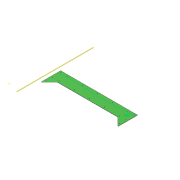
# Autodesk Inventor part: Acrylic-Side-Panel_CPY
Saved by Autodesk Inventor 2017 (Build 210142000, 142)
## iProperties
Created: 2016-07-12
Part Number: Acrylic-Side-Panel_CPY
Material: Generic
Document SubType Name: Modeling
Designer: joshmamo
Density: 1 g/cm^3
Appearance: Default
Author: joshmamo
Autodesk Inventor part; units mm, degrees
(part 1 of 3)
ref_plane "YZ Plane" through (0, 0, 0) normal (1, 0, 0) x (0, 1, 0)
ref_plane "XZ Plane" through (0, 0, 0) normal (0, 1, 0) x (-1, 0, 0)
ref_plane "XY Plane" through (0, 0, 0) normal (0, 0, 1) x (1, 0, 0)
ref_plane "Work Plane1" through (87.4375, 600, -660) normal (0, 0, -1) x (1, 0, 0)
sketch "Sketch1" plane through (87.4375, 600, -660) normal (0, 0, -1) x (1, 0, 0)
  line L0 (35.8425, 447.4613) -> (35.8425, 283.4613)
  line L1 (35.8425, 283.4613) -> (695.8425, 283.4613)
  line L2 (695.8425, 283.4613) -> (695.8425, 447.4613)
  line L3 (695.8425, 447.4613) -> (695.8027, 447.8653)
  line L4 (695.8027, 447.8653) -> (695.6848, 448.2538)
  line L5 (695.6848, 448.2538) -> (695.4935, 448.6119)
  line L6 (695.4935, 448.6119) -> (695.2359, 448.9257)
  line L7 (695.2359, 448.9257) -> (694.9221, 449.1833)
  line L8 (694.9221, 449.1833) -> (694.564, 449.3747)
  line L9 (694.564, 449.3747) -> (694.1755, 449.4925)
  line L10 (694.1755, 449.4925) -> (693.7714, 449.5323)
  line L11 (693.7714, 449.5323) -> (693.3674, 449.4925)
  line L12 (693.3674, 449.4925) -> (692.9789, 449.3747)
  line L13 (692.9789, 449.3747) -> (692.6208, 449.1833)
  line L14 (692.6208, 449.1833) -> (692.307, 448.9257)
  line L15 (692.307, 448.9257) -> (625.8425, 382.4613)
  line L16 (625.8425, 382.4613) -> (105.8425, 382.4613)
  line L17 (105.8425, 382.4613) -> (39.378, 448.9257)
  line L18 (39.378, 448.9257) -> (39.0642, 449.1833)
  line L19 (39.0642, 449.1833) -> (38.7061, 449.3747)
  line L20 (38.7061, 449.3747) -> (38.3176, 449.4925)
  line L21 (38.3176, 449.4925) -> (37.9136, 449.5323)
  line L22 (37.9136, 449.5323) -> (37.5095, 449.4925)
  line L23 (37.5095, 449.4925) -> (37.121, 449.3747)
  line L24 (37.121, 449.3747) -> (36.7629, 449.1833)
  line L25 (36.7629, 449.1833) -> (36.4491, 448.9257)
  line L26 (36.4491, 448.9257) -> (36.1915, 448.6119)
  line L27 (36.1915, 448.6119) -> (36.0002, 448.2538)
  line L28 (36.0002, 448.2538) -> (35.8823, 447.8653)
  line L29 (35.8823, 447.8653) -> (35.8425, 447.4613)
  line L30 (678.4084, 421.8091) -> (678.3225, 422.4613)
  line L31 (678.3225, 422.4613) -> (678.4084, 423.1135)
  line L32 (678.4084, 423.1135) -> (678.6601, 423.7213)
  line L33 (678.6601, 423.7213) -> (679.0606, 424.2432)
  line L34 (679.0606, 424.2432) -> (679.5825, 424.6437)
  line L35 (679.5825, 424.6437) -> (680.1903, 424.8954)
  line L36 (680.1903, 424.8954) -> (680.8425, 424.9813)
  line L37 (680.8425, 424.9813) -> (681.4947, 424.8954)
  line L38 (681.4947, 424.8954) -> (682.1025, 424.6437)
  line L39 (682.1025, 424.6437) -> (682.6244, 424.2432)
  line L40 (682.6244, 424.2432) -> (683.0249, 423.7213)
  line L41 (683.0249, 423.7213) -> (683.2766, 423.1135)
  line L42 (683.2766, 423.1135) -> (683.3625, 422.4613)
  line L43 (683.3625, 422.4613) -> (683.2766, 421.8091)
  line L44 (683.2766, 421.8091) -> (683.0249, 421.2013)
  line L45 (683.0249, 421.2013) -> (682.6244, 420.6794)
  line L46 (682.6244, 420.6794) -> (682.1025, 420.2789)
  line L47 (682.1025, 420.2789) -> (681.4947, 420.0271)
  line L48 (681.4947, 420.0271) -> (680.8425, 419.9413)
  line L49 (680.8425, 419.9413) -> (680.1903, 420.0271)
  line L50 (680.1903, 420.0271) -> (679.5825, 420.2789)
  line L51 (679.5825, 420.2789) -> (679.0606, 420.6794)
  line L52 (679.0606, 420.6794) -> (678.6601, 421.2013)
  line L53 (678.6601, 421.2013) -> (678.4084, 421.8091)
  line L54 (103.6601, 368.7213) -> (104.0606, 369.2432)
  line L55 (104.0606, 369.2432) -> (104.5825, 369.6437)
  line L56 (104.5825, 369.6437) -> (105.1903, 369.8954)
  line L57 (105.1903, 369.8954) -> (105.8425, 369.9813)
  line L58 (105.8425, 369.9813) -> (106.4947, 369.8954)
  line L59 (106.4947, 369.8954) -> (107.1025, 369.6437)
  line L60 (107.1025, 369.6437) -> (107.6244, 369.2432)
  line L61 (107.6244, 369.2432) -> (108.0249, 368.7213)
  line L62 (108.0249, 368.7213) -> (108.2766, 368.1135)
  line L63 (108.2766, 368.1135) -> (108.3625, 367.4613)
  line L64 (108.3625, 367.4613) -> (108.2766, 366.8091)
  line L65 (108.2766, 366.8091) -> (108.0249, 366.2013)
  line L66 (108.0249, 366.2013) -> (107.6244, 365.6794)
  line L67 (107.6244, 365.6794) -> (107.1025, 365.2789)
  line L68 (107.1025, 365.2789) -> (106.4947, 365.0271)
  line L69 (106.4947, 365.0271) -> (105.8425, 364.9413)
  line L70 (105.8425, 364.9413) -> (105.1903, 365.0271)
  line L71 (105.1903, 365.0271) -> (104.5825, 365.2789)
  line L72 (104.5825, 365.2789) -> (104.0606, 365.6794)
  line L73 (104.0606, 365.6794) -> (103.6601, 366.2013)
  line L74 (103.6601, 366.2013) -> (103.4084, 366.8091)
  line L75 (103.4084, 366.8091) -> (103.3225, 367.4613)
  line L76 (103.3225, 367.4613) -> (103.4084, 368.1135)
  line L77 (103.4084, 368.1135) -> (103.6601, 368.7213)
  line L78 (235.1106, 369.2432) -> (235.6325, 369.6437)
  line L79 (235.6325, 369.6437) -> (236.2403, 369.8954)
  line L80 (236.2403, 369.8954) -> (236.8925, 369.9813)
  line L81 (236.8925, 369.9813) -> (237.5447, 369.8954)
  line L82 (237.5447, 369.8954) -> (238.1525, 369.6437)
  line L83 (238.1525, 369.6437) -> (238.6744, 369.2432)
  line L84 (238.6744, 369.2432) -> (239.0749, 368.7213)
  line L85 (239.0749, 368.7213) -> (239.3266, 368.1135)
  line L86 (239.3266, 368.1135) -> (239.4125, 367.4613)
  line L87 (239.4125, 367.4613) -> (239.3266, 366.8091)
  line L88 (239.3266, 366.8091) -> (239.0749, 366.2013)
  line L89 (239.0749, 366.2013) -> (238.6744, 365.6794)
  line L90 (238.6744, 365.6794) -> (238.1525, 365.2789)
  line L91 (238.1525, 365.2789) -> (237.5447, 365.0271)
  line L92 (237.5447, 365.0271) -> (236.8925, 364.9413)
  line L93 (236.8925, 364.9413) -> (236.2403, 365.0271)
  line L94 (236.2403, 365.0271) -> (235.6325, 365.2789)
  line L95 (235.6325, 365.2789) -> (235.1106, 365.6794)
  line L96 (235.1106, 365.6794) -> (234.7101, 366.2013)
  line L97 (234.7101, 366.2013) -> (234.4584, 366.8091)
  line L98 (234.4584, 366.8091) -> (234.3725, 367.4613)
  line L99 (234.3725, 367.4613) -> (234.4584, 368.1135)
  line L100 (234.4584, 368.1135) -> (234.7101, 368.7213)
  line L101 (234.7101, 368.7213) -> (235.1106, 369.2432)
  line L102 (363.4084, 366.8091) -> (363.3225, 367.4613)
  line L103 (363.3225, 367.4613) -> (363.4084, 368.1135)
  line L104 (363.4084, 368.1135) -> (363.6601, 368.7213)
  line L105 (363.6601, 368.7213) -> (364.0606, 369.2432)
  line L106 (364.0606, 369.2432) -> (364.5825, 369.6437)
  line L107 (364.5825, 369.6437) -> (365.1903, 369.8954)
  line L108 (365.1903, 369.8954) -> (365.8425, 369.9813)
  line L109 (365.8425, 369.9813) -> (366.4947, 369.8954)
  line L110 (366.4947, 369.8954) -> (367.1025, 369.6437)
  line L111 (367.1025, 369.6437) -> (367.6244, 369.2432)
  line L112 (367.6244, 369.2432) -> (368.0249, 368.7213)
  line L113 (368.0249, 368.7213) -> (368.2766, 368.1135)
  line L114 (368.2766, 368.1135) -> (368.3625, 367.4613)
  line L115 (368.3625, 367.4613) -> (368.2766, 366.8091)
  line L116 (368.2766, 366.8091) -> (368.0249, 366.2013)
  line L117 (368.0249, 366.2013) -> (367.6244, 365.6794)
  line L118 (367.6244, 365.6794) -> (367.1025, 365.2789)
  line L119 (367.1025, 365.2789) -> (366.4947, 365.0271)
  line L120 (366.4947, 365.0271) -> (365.8425, 364.9413)
  line L121 (365.8425, 364.9413) -> (365.1903, 365.0271)
  line L122 (365.1903, 365.0271) -> (364.5825, 365.2789)
  line L123 (364.5825, 365.2789) -> (364.0606, 365.6794)
  line L124 (364.0606, 365.6794) -> (363.6601, 366.2013)
  line L125 (363.6601, 366.2013) -> (363.4084, 366.8091)
  line L126 (492.3584, 366.8091) -> (492.2725, 367.4613)
  line L127 (492.2725, 367.4613) -> (492.3584, 368.1135)
  line L128 (492.3584, 368.1135) -> (492.6101, 368.7213)
  line L129 (492.6101, 368.7213) -> (493.0106, 369.2432)
  line L130 (493.0106, 369.2432) -> (493.5325, 369.6437)
  line L131 (493.5325, 369.6437) -> (494.1403, 369.8954)
  line L132 (494.1403, 369.8954) -> (494.7925, 369.9813)
  line L133 (494.7925, 369.9813) -> (495.4447, 369.8954)
  line L134 (495.4447, 369.8954) -> (496.0525, 369.6437)
  line L135 (496.0525, 369.6437) -> (496.5744, 369.2432)
  line L136 (496.5744, 369.2432) -> (496.9749, 368.7213)
  line L137 (496.9749, 368.7213) -> (497.2266, 368.1135)
  line L138 (497.2266, 368.1135) -> (497.3125, 367.4613)
  line L139 (497.3125, 367.4613) -> (497.2266, 366.8091)
  line L140 (497.2266, 366.8091) -> (496.9749, 366.2013)
  line L141 (496.9749, 366.2013) -> (496.5744, 365.6794)
  line L142 (496.5744, 365.6794) -> (496.0525, 365.2789)
  line L143 (496.0525, 365.2789) -> (495.4447, 365.0271)
  line L144 (495.4447, 365.0271) -> (494.7925, 364.9413)
  line L145 (494.7925, 364.9413) -> (494.1403, 365.0271)
  line L146 (494.1403, 365.0271) -> (493.5325, 365.2789)
  line L147 (493.5325, 365.2789) -> (493.0106, 365.6794)
  line L148 (493.0106, 365.6794) -> (492.6101, 366.2013)
  line L149 (492.6101, 366.2013) -> (492.3584, 366.8091)
  line L150 (48.4084, 296.809) -> (48.3225, 297.4613)
  line L151 (48.3225, 297.4613) -> (48.4084, 298.1135)
  line L152 (48.4084, 298.1135) -> (48.6601, 298.7212)
  line L153 (48.6601, 298.7212) -> (49.0606, 299.2432)
  line L154 (49.0606, 299.2432) -> (49.5825, 299.6437)
  line L155 (49.5825, 299.6437) -> (50.1903, 299.8954)
  line L156 (50.1903, 299.8954) -> (50.8425, 299.9813)
  line L157 (50.8425, 299.9813) -> (51.4947, 299.8954)
  line L158 (51.4947, 299.8954) -> (52.1025, 299.6437)
  line L159 (52.1025, 299.6437) -> (52.6244, 299.2432)
  line L160 (52.6244, 299.2432) -> (53.0249, 298.7212)
  line L161 (53.0249, 298.7212) -> (53.2766, 298.1135)
  line L162 (53.2766, 298.1135) -> (53.3625, 297.4613)
  line L163 (53.3625, 297.4613) -> (53.2766, 296.809)
  line L164 (53.2766, 296.809) -> (53.0249, 296.2012)
  line L165 (53.0249, 296.2012) -> (52.6244, 295.6793)
  line L166 (52.6244, 295.6793) -> (52.1025, 295.2789)
  line L167 (52.1025, 295.2789) -> (51.4947, 295.0271)
  line L168 (51.4947, 295.0271) -> (50.8425, 294.9413)
  line L169 (50.8425, 294.9413) -> (50.1903, 295.0271)
  line L170 (50.1903, 295.0271) -> (49.5825, 295.2789)
  line L171 (49.5825, 295.2789) -> (49.0606, 295.6793)
  line L172 (49.0606, 295.6793) -> (48.6601, 296.2012)
  line L173 (48.6601, 296.2012) -> (48.4084, 296.809)
  line L174 (48.4084, 366.8091) -> (48.3225, 367.4613)
  line L175 (48.3225, 367.4613) -> (48.4084, 368.1135)
  line L176 (48.4084, 368.1135) -> (48.6601, 368.7213)
  line L177 (48.6601, 368.7213) -> (49.0606, 369.2432)
  line L178 (49.0606, 369.2432) -> (49.5825, 369.6437)
  line L179 (49.5825, 369.6437) -> (50.1903, 369.8954)
  line L180 (50.1903, 369.8954) -> (50.8425, 369.9813)
  line L181 (50.8425, 369.9813) -> (51.4947, 369.8954)
  line L182 (51.4947, 369.8954) -> (52.1025, 369.6437)
  line L183 (52.1025, 369.6437) -> (52.6244, 369.2432)
  line L184 (52.6244, 369.2432) -> (53.0249, 368.7213)
  line L185 (53.0249, 368.7213) -> (53.2766, 368.1135)
  line L186 (53.2766, 368.1135) -> (53.3625, 367.4613)
  line L187 (53.3625, 367.4613) -> (53.2766, 366.8091)
  line L188 (53.2766, 366.8091) -> (53.0249, 366.2013)
  line L189 (53.0249, 366.2013) -> (52.6244, 365.6794)
  line L190 (52.6244, 365.6794) -> (52.1025, 365.2789)
  line L191 (52.1025, 365.2789) -> (51.4947, 365.0271)
  line L192 (51.4947, 365.0271) -> (50.8425, 364.9413)
  line L193 (50.8425, 364.9413) -> (50.1903, 365.0271)
  line L194 (50.1903, 365.0271) -> (49.5825, 365.2789)
  line L195 (49.5825, 365.2789) -> (49.0606, 365.6794)
  line L196 (49.0606, 365.6794) -> (48.6601, 366.2013)
  line L197 (48.6601, 366.2013) -> (48.4084, 366.8091)
  line L198 (48.4084, 421.8091) -> (48.3225, 422.4613)
  line L199 (48.3225, 422.4613) -> (48.4084, 423.1135)
  line L200 (48.4084, 423.1135) -> (48.6601, 423.7213)
  line L201 (48.6601, 423.7213) -> (49.0606, 424.2432)
  line L202 (49.0606, 424.2432) -> (49.5825, 424.6437)
  line L203 (49.5825, 424.6437) -> (50.1903, 424.8954)
  line L204 (50.1903, 424.8954) -> (50.8425, 424.9813)
  line L205 (50.8425, 424.9813) -> (51.4947, 424.8954)
  line L206 (51.4947, 424.8954) -> (52.1025, 424.6437)
  line L207 (52.1025, 424.6437) -> (52.6244, 424.2432)
  line L208 (52.6244, 424.2432) -> (53.0249, 423.7213)
  line L209 (53.0249, 423.7213) -> (53.2766, 423.1135)
  line L210 (53.2766, 423.1135) -> (53.3625, 422.4613)
  line L211 (53.3625, 422.4613) -> (53.2766, 421.8091)
  line L212 (53.2766, 421.8091) -> (53.0249, 421.2013)
  line L213 (53.0249, 421.2013) -> (52.6244, 420.6794)
  line L214 (52.6244, 420.6794) -> (52.1025, 420.2789)
  line L215 (52.1025, 420.2789) -> (51.4947, 420.0271)
  line L216 (51.4947, 420.0271) -> (50.8425, 419.9413)
  line L217 (50.8425, 419.9413) -> (50.1903, 420.0271)
  line L218 (50.1903, 420.0271) -> (49.5825, 420.2789)
  line L219 (49.5825, 420.2789) -> (49.0606, 420.6794)
  line L220 (49.0606, 420.6794) -> (48.6601, 421.2013)
  line L221 (48.6601, 421.2013) -> (48.4084, 421.8091)
  line L222 (678.4084, 366.8091) -> (678.3225, 367.4613)
  line L223 (678.3225, 367.4613) -> (678.4084, 368.1135)
  line L224 (678.4084, 368.1135) -> (678.6601, 368.7213)
  line L225 (678.6601, 368.7213) -> (679.0606, 369.2432)
  line L226 (679.0606, 369.2432) -> (679.5825, 369.6437)
  line L227 (679.5825, 369.6437) -> (680.1903, 369.8954)
  line L228 (680.1903, 369.8954) -> (680.8425, 369.9813)
  line L229 (680.8425, 369.9813) -> (681.4947, 369.8954)
  line L230 (681.4947, 369.8954) -> (682.1025, 369.6437)
  line L231 (682.1025, 369.6437) -> (682.6244, 369.2432)
  line L232 (682.6244, 369.2432) -> (683.0249, 368.7213)
  line L233 (683.0249, 368.7213) -> (683.2766, 368.1135)
  line L234 (683.2766, 368.1135) -> (683.3625, 367.4613)
  line L235 (683.3625, 367.4613) -> (683.2766, 366.8091)
  line L236 (683.2766, 366.8091) -> (683.0249, 366.2013)
  line L237 (683.0249, 366.2013) -> (682.6244, 365.6794)
  line L238 (682.6244, 365.6794) -> (682.1025, 365.2789)
  line L239 (682.1025, 365.2789) -> (681.4947, 365.0271)
  line L240 (681.4947, 365.0271) -> (680.8425, 364.9413)
  line L241 (680.8425, 364.9413) -> (680.1903, 365.0271)
  line L242 (680.1903, 365.0271) -> (679.5825, 365.2789)
  line L243 (679.5825, 365.2789) -> (679.0606, 365.6794)
  line L244 (679.0606, 365.6794) -> (678.6601, 366.2013)
  line L245 (678.6601, 366.2013) -> (678.4084, 366.8091)
  line L246 (680.1903, 295.0271) -> (679.5825, 295.2789)
  line L247 (679.5825, 295.2789) -> (679.0606, 295.6793)
  line L248 (679.0606, 295.6793) -> (678.6601, 296.2012)
  line L249 (678.6601, 296.2012) -> (678.4084, 296.809)
  line L250 (678.4084, 296.809) -> (678.3225, 297.4613)
  line L251 (678.3225, 297.4613) -> (678.4084, 298.1135)
  line L252 (678.4084, 298.1135) -> (678.6601, 298.7212)
  line L253 (678.6601, 298.7212) -> (679.0606, 299.2432)
  line L254 (679.0606, 299.2432) -> (679.5825, 299.6437)
  line L255 (679.5825, 299.6437) -> (680.1903, 299.8954)
  line L256 (680.1903, 299.8954) -> (680.8425, 299.9813)
  line L257 (680.8425, 299.9813) -> (681.4947, 299.8954)
  line L258 (681.4947, 299.8954) -> (682.1025, 299.6437)
  line L259 (682.1025, 299.6437) -> (682.6244, 299.2432)
  line L260 (682.6244, 299.2432) -> (683.0249, 298.7212)
  line L261 (683.0249, 298.7212) -> (683.2766, 298.1135)
  line L262 (683.2766, 298.1135) -> (683.3625, 297.4613)
  line L263 (683.3625, 297.4613) -> (683.2766, 296.809)
  line L264 (683.2766, 296.809) -> (683.0249, 296.2012)
  line L265 (683.0249, 296.2012) -> (682.6244, 295.6793)
  line L266 (682.6244, 295.6793) -> (682.1025, 295.2789)
  line L267 (682.1025, 295.2789) -> (681.4947, 295.0271)
  line L268 (681.4947, 295.0271) -> (680.8425, 294.9413)
  line L269 (680.8425, 294.9413) -> (680.1903, 295.0271)
  line L270 (623.4084, 296.809) -> (623.3225, 297.4613)
  line L271 (623.3225, 297.4613) -> (623.4084, 298.1135)
  line L272 (623.4084, 298.1135) -> (623.6601, 298.7212)
  line L273 (623.6601, 298.7212) -> (624.0606, 299.2432)
  line L274 (624.0606, 299.2432) -> (624.5825, 299.6437)
  line L275 (624.5825, 299.6437) -> (625.1903, 299.8954)
  line L276 (625.1903, 299.8954) -> (625.8425, 299.9813)
  line L277 (625.8425, 299.9813) -> (626.4947, 299.8954)
  line L278 (626.4947, 299.8954) -> (627.1025, 299.6437)
  line L279 (627.1025, 299.6437) -> (627.6244, 299.2432)
  line L280 (627.6244, 299.2432) -> (628.0249, 298.7212)
  line L281 (628.0249, 298.7212) -> (628.2766, 298.1135)
  line L282 (628.2766, 298.1135) -> (628.3625, 297.4613)
  line L283 (628.3625, 297.4613) -> (628.2766, 296.809)
  line L284 (628.2766, 296.809) -> (628.0249, 296.2012)
  line L285 (628.0249, 296.2012) -> (627.6244, 295.6793)
  line L286 (627.6244, 295.6793) -> (627.1025, 295.2789)
  line L287 (627.1025, 295.2789) -> (626.4947, 295.0271)
  line L288 (626.4947, 295.0271) -> (625.8425, 294.9413)
  line L289 (625.8425, 294.9413) -> (625.1903, 295.0271)
  line L290 (625.1903, 295.0271) -> (624.5825, 295.2789)
  line L291 (624.5825, 295.2789) -> (624.0606, 295.6793)
  line L292 (624.0606, 295.6793) -> (623.6601, 296.2012)
  line L293 (623.6601, 296.2012) -> (623.4084, 296.809)
  line L294 (623.4084, 366.8091) -> (623.3225, 367.4613)
  line L295 (623.3225, 367.4613) -> (623.4084, 368.1135)
  line L296 (623.4084, 368.1135) -> (623.6601, 368.7213)
  line L297 (623.6601, 368.7213) -> (624.0606, 369.2432)
  line L298 (624.0606, 369.2432) -> (624.5825, 369.6437)
  line L299 (624.5825, 369.6437) -> (625.1903, 369.8954)
  line L300 (625.1903, 369.8954) -> (625.8425, 369.9813)
  line L301 (625.8425, 369.9813) -> (626.4947, 369.8954)
  line L302 (626.4947, 369.8954) -> (627.1025, 369.6437)
  line L303 (627.1025, 369.6437) -> (627.6244, 369.2432)
  line L304 (627.6244, 369.2432) -> (628.0249, 368.7213)
  line L305 (628.0249, 368.7213) -> (628.2766, 368.1135)
  line L306 (628.2766, 368.1135) -> (628.3625, 367.4613)
  line L307 (628.3625, 367.4613) -> (628.2766, 366.8091)
  line L308 (628.2766, 366.8091) -> (628.0249, 366.2013)
  line L309 (628.0249, 366.2013) -> (627.6244, 365.6794)
  line L310 (627.6244, 365.6794) -> (627.1025, 365.2789)
  line L311 (627.1025, 365.2789) -> (626.4947, 365.0271)
  line L312 (626.4947, 365.0271) -> (625.8425, 364.9413)
  line L313 (625.8425, 364.9413) -> (625.1903, 365.0271)
  line L314 (625.1903, 365.0271) -> (624.5825, 365.2789)
  line L315 (624.5825, 365.2789) -> (624.0606, 365.6794)
  line L316 (624.0606, 365.6794) -> (623.6601, 366.2013)
  line L317 (623.6601, 366.2013) -> (623.4084, 366.8091)
  line L318 (492.3584, 296.809) -> (492.2725, 297.4613)
  line L319 (492.2725, 297.4613) -> (492.3584, 298.1135)
  line L320 (492.3584, 298.1135) -> (492.6101, 298.7212)
  line L321 (492.6101, 298.7212) -> (493.0106, 299.2432)
  line L322 (493.0106, 299.2432) -> (493.5325, 299.6437)
  line L323 (493.5325, 299.6437) -> (494.1403, 299.8954)
  line L324 (494.1403, 299.8954) -> (494.7925, 299.9813)
  line L325 (494.7925, 299.9813) -> (495.4447, 299.8954)
  line L326 (495.4447, 299.8954) -> (496.0525, 299.6437)
  line L327 (496.0525, 299.6437) -> (496.5744, 299.2432)
  line L328 (496.5744, 299.2432) -> (496.9749, 298.7212)
  line L329 (496.9749, 298.7212) -> (497.2266, 298.1135)
  line L330 (497.2266, 298.1135) -> (497.3125, 297.4613)
  line L331 (497.3125, 297.4613) -> (497.2266, 296.809)
  line L332 (497.2266, 296.809) -> (496.9749, 296.2012)
  line L333 (496.9749, 296.2012) -> (496.5744, 295.6793)
  line L334 (496.5744, 295.6793) -> (496.0525, 295.2789)
  line L335 (496.0525, 295.2789) -> (495.4447, 295.0271)
  line L336 (495.4447, 295.0271) -> (494.7925, 294.9413)
  line L337 (494.7925, 294.9413) -> (494.1403, 295.0271)
  line L338 (494.1403, 295.0271) -> (493.5325, 295.2789)
  line L339 (493.5325, 295.2789) -> (493.0106, 295.6793)
  line L340 (493.0106, 295.6793) -> (492.6101, 296.2012)
  line L341 (492.6101, 296.2012) -> (492.3584, 296.809)
  line L342 (363.4084, 296.809) -> (363.3225, 297.4613)
  line L343 (363.3225, 297.4613) -> (363.4084, 298.1135)
  line L344 (363.4084, 298.1135) -> (363.6601, 298.7212)
  line L345 (363.6601, 298.7212) -> (364.0606, 299.2432)
  line L346 (364.0606, 299.2432) -> (364.5825, 299.6437)
  line L347 (364.5825, 299.6437) -> (365.1903, 299.8954)
  line L348 (365.1903, 299.8954) -> (365.8425, 299.9813)
  line L349 (365.8425, 299.9813) -> (366.4947, 299.8954)
  line L350 (366.4947, 299.8954) -> (367.1025, 299.6437)
  line L351 (367.1025, 299.6437) -> (367.6244, 299.2432)
  line L352 (367.6244, 299.2432) -> (368.0249, 298.7212)
  line L353 (368.0249, 298.7212) -> (368.2766, 298.1135)
  line L354 (368.2766, 298.1135) -> (368.3625, 297.4613)
  line L355 (368.3625, 297.4613) -> (368.2766, 296.809)
  line L356 (368.2766, 296.809) -> (368.0249, 296.2012)
  line L357 (368.0249, 296.2012) -> (367.6244, 295.6793)
  line L358 (367.6244, 295.6793) -> (367.1025, 295.2789)
  line L359 (367.1025, 295.2789) -> (366.4947, 295.0271)
  line L360 (366.4947, 295.0271) -> (365.8425, 294.9413)
  line L361 (365.8425, 294.9413) -> (365.1903, 295.0271)
  line L362 (365.1903, 295.0271) -> (364.5825, 295.2789)
  line L363 (364.5825, 295.2789) -> (364.0606, 295.6793)
  line L364 (364.0606, 295.6793) -> (363.6601, 296.2012)
  line L365 (363.6601, 296.2012) -> (363.4084, 296.809)
  line L366 (108.0249, 296.2012) -> (107.6244, 295.6793)
  line L367 (107.6244, 295.6793) -> (107.1025, 295.2789)
  line L368 (107.1025, 295.2789) -> (106.4947, 295.0271)
  line L369 (106.4947, 295.0271) -> (105.8425, 294.9413)
  line L370 (105.8425, 294.9413) -> (105.1903, 295.0271)
  line L371 (105.1903, 295.0271) -> (104.5825, 295.2789)
  line L372 (104.5825, 295.2789) -> (104.0606, 295.6793)
  line L373 (104.0606, 295.6793) -> (103.6601, 296.2012)
  line L374 (103.6601, 296.2012) -> (103.4084, 296.809)
  line L375 (103.4084, 296.809) -> (103.3225, 297.4613)
  line L376 (103.3225, 297.4613) -> (103.4084, 298.1135)
  line L377 (103.4084, 298.1135) -> (103.6601, 298.7212)
  line L378 (103.6601, 298.7212) -> (104.0606, 299.2432)
  line L379 (104.0606, 299.2432) -> (104.5825, 299.6437)
  line L380 (104.5825, 299.6437) -> (105.1903, 299.8954)
  line L381 (105.1903, 299.8954) -> (105.8425, 299.9813)
  line L382 (105.8425, 299.9813) -> (106.4947, 299.8954)
  line L383 (106.4947, 299.8954) -> (107.1025, 299.6437)
  line L384 (107.1025, 299.6437) -> (107.6244, 299.2432)
  line L385 (107.6244, 299.2432) -> (108.0249, 298.7212)
  line L386 (108.0249, 298.7212) -> (108.2766, 298.1135)
  line L387 (108.2766, 298.1135) -> (108.3625, 297.4613)
  line L388 (108.3625, 297.4613) -> (108.2766, 296.809)
  line L389 (108.2766, 296.809) -> (108.0249, 296.2012)
  line L390 (234.7101, 296.2012) -> (234.4584, 296.809)
  line L391 (234.4584, 296.809) -> (234.3725, 297.4613)
  line L392 (234.3725, 297.4613) -> (234.4584, 298.1135)
  line L393 (234.4584, 298.1135) -> (234.7101, 298.7212)
  line L394 (234.7101, 298.7212) -> (235.1106, 299.2432)
  line L395 (235.1106, 299.2432) -> (235.6325, 299.6437)
  line L396 (235.6325, 299.6437) -> (236.2403, 299.8954)
  line L397 (236.2403, 299.8954) -> (236.8925, 299.9813)
  line L398 (236.8925, 299.9813) -> (237.5447, 299.8954)
  line L399 (237.5447, 299.8954) -> (238.1525, 299.6437)
  line L400 (238.1525, 299.6437) -> (238.6744, 299.2432)
  line L401 (238.6744, 299.2432) -> (239.0749, 298.7212)
  line L402 (239.0749, 298.7212) -> (239.3266, 298.1135)
  line L403 (239.3266, 298.1135) -> (239.4125, 297.4613)
  line L404 (239.4125, 297.4613) -> (239.3266, 296.809)
  line L405 (239.3266, 296.809) -> (239.0749, 296.2012)
  line L406 (239.0749, 296.2012) -> (238.6744, 295.6793)
  line L407 (238.6744, 295.6793) -> (238.1525, 295.2789)
  line L408 (238.1525, 295.2789) -> (237.5447, 295.0271)
  line L409 (237.5447, 295.0271) -> (236.8925, 294.9413)
  line L410 (236.8925, 294.9413) -> (236.2403, 295.0271)
  line L411 (236.2403, 295.0271) -> (235.6325, 295.2789)
  line L412 (235.6325, 295.2789) -> (235.1106, 295.6793)
  line L413 (235.1106, 295.6793) -> (234.7101, 296.2012)
  line L414 (695.8306, 295.4812) -> (679.2642, 301.1207)
  line L415 (679.2642, 301.1207) -> (657.0353, 304.5772)
  line L416 (657.0353, 304.5772) -> (657.6968, 304.9548)
  line L417 (657.6968, 304.9548) -> (658.5282, 305.4982)
  line L418 (658.5282, 305.4982) -> (659.1348, 305.9757)
  line L419 (659.1348, 305.9757) -> (659.5991, 306.4507)
  line L420 (659.5991, 306.4507) -> (660.0336, 306.9385)
  line L421 (660.0336, 306.9385) -> (660.412, 307.476)
  line L422 (660.412, 307.476) -> (660.7697, 308.1634)
  line L423 (660.7697, 308.1634) -> (661.0511, 308.8919)
  line L424 (661.0511, 308.8919) -> (661.2395, 309.6349)
  line L425 (661.2395, 309.6349) -> (661.3351, 310.4377)
  line L426 (661.3351, 310.4377) -> (661.3351, 311.2803)
  line L427 (661.3351, 311.2803) -> (661.2419, 312.1649)
  line L428 (661.2419, 312.1649) -> (661.1668, 312.647)
  line L429 (661.1668, 312.647) -> (661.0779, 313.1154)
  line L430 (661.0779, 313.1154) -> (660.9514, 313.5705)
  line L431 (660.9514, 313.5705) -> (660.5889, 314.4761)
  line L432 (660.5889, 314.4761) -> (660.1076, 315.3361)
  line L433 (660.1076, 315.3361) -> (659.4705, 316.1087)
  line L434 (659.4705, 316.1087) -> (659.0302, 316.5716)
  line L435 (659.0302, 316.5716) -> (658.6188, 317.0424)
  line L436 (658.6188, 317.0424) -> (658.1951, 317.5012)
  line L437 (658.1951, 317.5012) -> (657.3719, 318.2996)
  line L438 (657.3719, 318.2996) -> (656.5243, 319.1068)
  line L439 (656.5243, 319.1068) -> (655.6986, 319.9347)
  line L440 (655.6986, 319.9347) -> (655.0956, 320.6675)
  line L441 (655.0956, 320.6675) -> (654.646, 321.4804)
  line L442 (654.646, 321.4804) -> (654.3821, 322.395)
  line L443 (654.3821, 322.395) -> (654.1985, 323.5381)
  line L444 (654.1985, 323.5381) -> (654.001, 324.689)
  line L445 (654.001, 324.689) -> (653.8148, 325.8415)
  line L446 (653.8148, 325.8415) -> (653.7946, 326.9904)
  line L447 (653.7946, 326.9904) -> (654.1438, 328.009)
  line L448 (654.1438, 328.009) -> (654.8868, 328.8853)
  line L449 (654.8868, 328.8853) -> (655.3734, 329.17)
  line L450 (655.3734, 329.17) -> (655.8563, 329.2702)
  line L451 (655.8563, 329.2702) -> (656.3521, 329.3194)
  line L452 (656.3521, 329.3194) -> (657.1162, 329.3041)
  line L453 (657.1162, 329.3041) -> (657.8638, 329.1118)
  line L454 (657.8638, 329.1118) -> (658.6053, 328.8757)
  line L455 (658.6053, 328.8757) -> (659.5177, 328.7178)
  line L456 (659.5177, 328.7178) -> (660.2065, 328.9029)
  line L457 (660.2065, 328.9029) -> (660.7407, 329.5226)
  line L458 (660.7407, 329.5226) -> (660.9024, 329.8038)
  line L459 (660.9024, 329.8038) -> (661.0472, 330.0253)
  line L460 (661.0472, 330.0253) -> (661.1926, 330.2463)
  line L461 (661.1926, 330.2463) -> (661.4272, 330.6177)
  line L462 (661.4272, 330.6177) -> (661.6696, 331.0037)
  line L463 (661.6696, 331.0037) -> (661.9064, 331.3928)
  line L464 (661.9064, 331.3928) -> (661.9754, 331.5287)
  line L465 (661.9754, 331.5287) -> (662.0077, 331.6489)
  line L466 (662.0077, 331.6489) -> (662.0087, 331.7644)
  line L467 (662.0087, 331.7644) -> (661.9564, 331.8145)
  line L468 (661.9564, 331.8145) -> (661.8395, 331.8456)
  line L469 (661.8395, 331.8456) -> (661.7136, 331.8576)
  line L470 (661.7136, 331.8576) -> (660.9949, 331.8461)
  line L471 (660.9949, 331.8461) -> (660.2066, 331.8289)
  line L472 (660.2066, 331.8289) -> (659.4197, 331.7926)
  line L473 (659.4197, 331.7926) -> (658.8836, 331.6509)
  line L474 (658.8836, 331.6509) -> (658.4917, 331.3249)
  line L475 (658.4917, 331.3249) -> (658.1598, 330.9189)
  line L476 (658.1598, 330.9189) -> (657.9688, 330.6607)
  line L477 (657.9688, 330.6607) -> (657.8039, 330.4149)
  line L478 (657.8039, 330.4149) -> (657.6304, 330.1765)
  line L479 (657.6304, 330.1765) -> (657.533, 330.0899)
  line L480 (657.533, 330.0899) -> (657.4183, 330.0454)
  line L481 (657.4183, 330.0454) -> (657.3067, 330.0384)
  line L482 (657.3067, 330.0384) -> (656.6261, 330.1494)
  line L483 (656.6261, 330.1494) -> (655.8643, 330.1558)
  line L484 (655.8643, 330.1558) -> (655.1028, 330.0554)
  line L485 (655.1028, 330.0554) -> (654.9076, 330.0201)
  line L486 (654.9076, 330.0201) -> (654.7783, 330.0071)
  line L487 (654.7783, 330.0071) -> (654.6117, 329.9912)
  line L488 (654.6117, 329.9912) -> (654.8175, 330.3123)
  line L489 (654.8175, 330.3123) -> (655.0625, 330.6558)
  line L490 (655.0625, 330.6558) -> (655.3061, 330.9713)
  line L491 (655.3061, 330.9713) -> (656.1248, 331.8169)
  line L492 (656.1248, 331.8169) -> (657.156, 332.5831)
  line L493 (657.156, 332.5831) -> (658.318, 333.1542)
  line L494 (658.318, 333.1542) -> (659.3238, 333.4917)
  line L495 (659.3238, 333.4917) -> (660.3103, 333.7204)
  line L496 (660.3103, 333.7204) -> (661.3258, 333.7711)
  line L497 (661.3258, 333.7711) -> (662.4865, 333.6051)
  line L498 (662.4865, 333.6051) -> (663.6036, 333.2479)
  line L499 (663.6036, 333.2479) -> (664.5983, 332.6035)
  line L500 (664.5983, 332.6035) -> (664.9593, 332.2049)
  line L501 (664.9593, 332.2049) -> (665.1684, 331.8371)
  line L502 (665.1684, 331.8371) -> (665.3138, 331.4448)
  line L503 (665.3138, 331.4448) -> (665.4909, 330.7248)
  line L504 (665.4909, 330.7248) -> (665.6251, 329.9298)
  line L505 (665.6251, 329.9298) -> (665.6224, 329.125)
  line L506 (665.6224, 329.125) -> (665.4669, 328.4201)
  line L507 (665.4669, 328.4201) -> (665.187, 327.7847)
  line L508 (665.187, 327.7847) -> (664.7572, 327.2273)
  line L509 (664.7572, 327.2273) -> (664.5426, 327.0547)
  line L510 (664.5426, 327.0547) -> (664.3658, 326.9806)
  line L511 (664.3658, 326.9806) -> (664.1797, 326.934)
  line L512 (664.1797, 326.934) -> (663.8115, 326.8777)
  line L513 (663.8115, 326.8777) -> (663.401, 326.8289)
  line L514 (663.401, 326.8289) -> (662.9896, 326.7872)
  line L515 (662.9896, 326.7872) -> (662.4812, 326.8615)
  line L516 (662.4812, 326.8615) -> (662.0566, 327.2139)
  line L517 (662.0566, 327.2139) -> (661.8248, 327.687)
  line L518 (661.8248, 327.687) -> (661.8033, 327.9452)
  line L519 (661.8033, 327.9452) -> (661.8564, 328.1269)
  line L520 (661.8564, 328.1269) -> (662.0091, 328.257)
  line L521 (662.0091, 328.257) -> (662.2273, 328.2983)
  line L522 (662.2273, 328.2983) -> (662.4282, 328.2191)
  line L523 (662.4282, 328.2191) -> (662.6173, 328.0066)
  line L524 (662.6173, 328.0066) -> (662.7384, 328.0554)
  line L525 (662.7384, 328.0554) -> (662.8362, 328.1811)
  line L526 (662.8362, 328.1811) -> (662.9286, 328.2999)
  line L527 (662.9286, 328.2999) -> (662.6905, 328.6003)
  line L528 (662.6905, 328.6003) -> (662.3447, 328.8007)
  line L529 (662.3447, 328.8007) -> (662.0062, 328.8245)
  line L530 (662.0062, 328.8245) -> (661.6781, 328.647)
  line L531 (661.6781, 328.647) -> (661.4225, 328.3077)
  line L532 (661.4225, 328.3077) -> (661.2971, 327.8867)
  line L533 (661.2971, 327.8867) -> (661.3902, 327.2099)
  line L534 (661.3902, 327.2099) -> (661.7659, 326.5156)
  line L535 (661.7659, 326.5156) -> (662.3371, 326.0681)
  line L536 (662.3371, 326.0681) -> (662.8833, 325.9589)
  line L537 (662.8833, 325.9589) -> (663.417, 325.9428)
  line L538 (663.417, 325.9428) -> (663.9488, 325.9879)
  line L539 (663.9488, 325.9879) -> (665.0512, 326.3286)
  line L540 (665.0512, 326.3286) -> (666.0126, 327.1175)
  line L541 (666.0126, 327.1175) -> (666.7314, 328.1943)
  line L542 (666.7314, 328.1943) -> (667.0518, 328.9966)
  line L543 (667.0518, 328.9966) -> (667.0476, 329.6629)
  line L544 (667.0476, 329.6629) -> (666.8808, 330.3227)
  line L545 (666.8808, 330.3227) -> (666.8071, 330.5645)
  line L546 (666.8071, 330.5645) -> (666.7943, 330.6833)
  line L547 (666.7943, 330.6833) -> (666.8137, 330.7793)
  line L548 (666.8137, 330.7793) -> (666.8974, 330.8509)
  line L549 (666.8974, 330.8509) -> (667.0247, 330.9049)
  line L550 (667.0247, 330.9049) -> (667.1765, 330.9587)
  line L551 (667.1765, 330.9587) -> (667.1956, 330.8177)
  line L552 (667.1956, 330.8177) -> (667.1728, 330.6449)
  line L553 (667.1728, 330.6449) -> (667.1535, 330.4966)
  line L554 (667.1535, 330.4966) -> (667.4051, 330.4402)
  line L555 (667.4051, 330.4402) -> (667.6583, 330.5287)
  line L556 (667.6583, 330.5287) -> (667.8332, 330.7594)
  line L557 (667.8332, 330.7594) -> (667.8912, 331.0519)
  line L558 (667.8912, 331.0519) -> (667.796, 331.3723)
  line L559 (667.796, 331.3723) -> (667.5862, 331.6164)
  line L560 (667.5862, 331.6164) -> (667.3088, 331.7163)
  line L561 (667.3088, 331.7163) -> (667.0146, 331.7726)
  line L562 (667.0146, 331.7726) -> (666.7189, 331.7866)
  line L563 (666.7189, 331.7866) -> (666.4378, 331.7896)
  line L564 (666.4378, 331.7896) -> (666.2126, 331.8743)
  line L565 (666.2126, 331.8743) -> (666.0418, 332.0332)
  line L566 (666.0418, 332.0332) -> (665.5217, 332.7208)
  line L567 (665.5217, 332.7208) -> (664.7244, 333.4193)
  line L568 (664.7244, 333.4193) -> (663.7811, 333.9282)
  line L569 (663.7811, 333.9282) -> (662.7025, 334.2818)
  line L570 (662.7025, 334.2818) -> (661.5891, 334.4843)
  line L571 (661.5891, 334.4843) -> (660.4566, 334.4788)
  line L572 (660.4566, 334.4788) -> (658.7636, 334.0937)
  line L573 (658.7636, 334.0937) -> (657.0091, 333.3143)
  line L574 (657.0091, 333.3143) -> (655.4641, 332.1395)
  line L575 (655.4641, 332.1395) -> (654.9004, 331.551)
  line L576 (654.9004, 331.551) -> (654.6694, 331.3278)
  line L577 (654.6694, 331.3278) -> (654.4345, 331.1078)
  line L578 (654.4345, 331.1078) -> (654.3597, 331.0396)
  line L579 (654.3597, 331.0396) -> (654.3421, 331.0398)
  line L580 (654.3421, 331.0398) -> (654.3077, 331.0411)
  line L581 (654.3077, 331.0411) -> (654.2898, 331.293)
  line L582 (654.2898, 331.293) -> (654.2826, 331.6555)
  line L583 (654.2826, 331.6555) -> (654.29, 332.0174)
  line L584 (654.29, 332.0174) -> (654.3704, 333.0787)
  line L585 (654.3704, 333.0787) -> (654.4058, 334.4512)
  line L586 (654.4058, 334.4512) -> (654.3299, 335.8231)
  line L587 (654.3299, 335.8231) -> (654.2159, 336.7091)
  line L588 (654.2159, 336.7091) -> (654.1283, 337.3734)
  line L589 (654.1283, 337.3734) -> (654.0409, 338.0376)
  line L590 (654.0409, 338.0376) -> (654.0138, 338.5209)
  line L591 (654.0138, 338.5209) -> (654.1636, 338.732)
  line L592 (654.1636, 338.732) -> (654.4604, 338.745)
  line L593 (654.4604, 338.745) -> (655.1447, 338.6328)
  line L594 (655.1447, 338.6328) -> (656.0396, 338.84)
  line L595 (656.0396, 338.84) -> (656.7321, 339.4323)
  line L596 (656.7321, 339.4323) -> (657.0296, 340.146)
  line L597 (657.0296, 340.146) -> (657.3302, 340.7766)
  line L598 (657.3302, 340.7766) -> (657.6481, 341.4017)
  line L599 (657.6481, 341.4017) -> (657.768, 341.6619)
  line L600 (657.768, 341.6619) -> (657.7814, 341.7436)
  line L601 (657.7814, 341.7436) -> (657.7744, 341.8219)
  line L602 (657.7744, 341.8219) -> (657.7436, 341.865)
  line L603 (657.7436, 341.865) -> (657.6731, 341.8827)
  line L604 (657.6731, 341.8827) -> (657.5906, 341.885)
  line L605 (657.5906, 341.885) -> (657.1706, 341.8131)
  line L606 (657.1706, 341.8131) -> (656.5674, 341.7022)
  line L607 (656.5674, 341.7022) -> (655.9627, 341.6037)
  line L608 (655.9627, 341.6037) -> (655.2426, 341.4862)
  line L609 (655.2426, 341.4862) -> (654.5478, 341.2102)
  line L610 (654.5478, 341.2102) -> (653.9853, 340.7087)
  line L611 (653.9853, 340.7087) -> (653.8039, 340.4378)
  line L612 (653.8039, 340.4378) -> (653.7656, 340.4044)
  line L613 (653.7656, 340.4044) -> (653.7234, 340.3727)
  line L614 (653.7234, 340.3727) -> (653.5587, 340.707)
  line L615 (653.5587, 340.707) -> (653.3283, 341.244)
  line L616 (653.3283, 341.244) -> (653.0918, 341.7719)
  line L617 (653.0918, 341.7719) -> (652.4323, 342.9638)
  line L618 (652.4323, 342.9638) -> (651.3075, 344.3331)
  line L619 (651.3075, 344.3331) -> (649.9215, 345.4538)
  line L620 (649.9215, 345.4538) -> (648.9081, 346.0522)
  line L621 (648.9081, 346.0522) -> (648.2003, 346.3982)
  line L622 (648.2003, 346.3982) -> (647.4574, 346.6606)
  line L623 (647.4574, 346.6606) -> (646.4794, 346.8055)
  line L624 (646.4794, 346.8055) -> (645.4404, 346.6429)
  line L625 (645.4404, 346.6429) -> (644.5722, 346.0647)
  line L626 (644.5722, 346.0647) -> (644.1487, 345.5176)
  line L627 (644.1487, 345.5176) -> (643.8524, 345.3143)
  line L628 (643.8524, 345.3143) -> (643.5181, 345.1957)
  line L629 (643.5181, 345.1957) -> (643.2971, 345.1364)
  line L630 (643.2971, 345.1364) -> (643.1583, 345.1053)
  line L631 (643.1583, 345.1053) -> (643.0319, 345.058)
  line L632 (643.0319, 345.058) -> (642.8335, 344.9411)
  line L633 (642.8335, 344.9411) -> (642.6102, 344.9457)
  line L634 (642.6102, 344.9457) -> (642.4031, 345.0666)
  line L635 (642.4031, 345.0666) -> (642.2402, 345.1733)
  line L636 (642.2402, 345.1733) -> (642.0902, 345.2202)
  line L637 (642.0902, 345.2202) -> (641.9303, 345.2503)
  line L638 (641.9303, 345.2503) -> (641.7807, 345.2743)
  line L639 (641.7807, 345.2743) -> (641.6333, 345.2838)
  line L640 (641.6333, 345.2838) -> (641.4893, 345.3018)
  line L641 (641.4893, 345.3018) -> (641.2662, 345.3591)
  line L642 (641.2662, 345.3591) -> (641.0306, 345.3295)
  line L643 (641.0306, 345.3295) -> (640.8432, 345.1689)
  line L644 (640.8432, 345.1689) -> (640.7408, 345.0236)
  line L645 (640.7408, 345.0236) -> (640.6392, 344.9767)
  line L646 (640.6392, 344.9767) -> (640.5191, 344.9534)
  line L647 (640.5191, 344.9534) -> (640.423, 344.9582)
  line L648 (640.423, 344.9582) -> (640.3376, 344.9984)
  line L649 (640.3376, 344.9984) -> (640.2513, 345.0491)
  line L650 (640.2513, 345.0491) -> (640.0332, 345.1232)
  line L651 (640.0332, 345.1232) -> (639.767, 345.1076)
  line L652 (639.767, 345.1076) -> (639.5404, 344.9501)
  line L653 (639.5404, 344.9501) -> (639.3557, 344.7238)
  line L654 (639.3557, 344.7238) -> (639.1739, 344.5264)
  line L655 (639.1739, 344.5264) -> (638.9705, 344.3188)
  line L656 (638.9705, 344.3188) -> (638.9733, 344.1462)
  line L657 (638.9733, 344.1462) -> (639.1451, 344.017)
  line L658 (639.1451, 344.017) -> (639.327, 343.8801)
  line L659 (639.327, 343.8801) -> (639.3634, 343.671)
  line L660 (639.3634, 343.671) -> (639.2626, 343.3877)
  line L661 (639.2626, 343.3877) -> (639.1519, 343.0763)
  line L662 (639.1519, 343.0763) -> (638.7812, 343.0288)
  line L663 (638.7812, 343.0288) -> (638.3423, 343.3863)
  line L664 (638.3423, 343.3863) -> (637.9434, 343.8002)
  line L665 (637.9434, 343.8002) -> (637.7296, 343.8631)
  line L666 (637.7296, 343.8631) -> (637.7233, 343.7047)
  line L667 (637.7233, 343.7047) -> (637.727, 343.5525)
  line L668 (637.727, 343.5525) -> (637.7704, 343.3349)
  line L669 (637.7704, 343.3349) -> (637.8307, 343.0596)
  line L670 (637.8307, 343.0596) -> (637.8234, 342.7786)
  line L671 (637.8234, 342.7786) -> (637.7695, 342.6068)
  line L672 (637.7695, 342.6068) -> (637.7947, 342.5173)
  line L673 (637.7947, 342.5173) -> (637.8473, 342.4249)
  line L674 (637.8473, 342.4249) -> (637.9848, 342.2212)
  line L675 (637.9848, 342.2212) -> (638.0713, 341.8944)
  line L676 (638.0713, 341.8944) -> (638.0525, 341.5453)
  line L677 (638.0525, 341.5453) -> (637.9611, 340.8865)
  line L678 (637.9611, 340.8865) -> (637.9916, 339.9972)
  line L679 (637.9916, 339.9972) -> (638.3688, 339.2047)
  line L680 (638.3688, 339.2047) -> (638.9016, 338.76)
  line L681 (638.9016, 338.76) -> (639.2596, 338.5571)
  line L682 (639.2596, 338.5571) -> (639.6267, 338.3665)
  line L683 (639.6267, 338.3665) -> (639.8959, 338.2197)
  line L684 (639.8959, 338.2197) -> (640.078, 338.1171)
  line L685 (640.078, 338.1171) -> (640.2676, 338.0095)
  line L686 (640.2676, 338.0095) -> (640.5028, 338.03)
  line L687 (640.5028, 338.03) -> (640.6816, 338.0539)
  line L688 (640.6816, 338.0539) -> (640.8096, 337.8945)
  line L689 (640.8096, 337.8945) -> (640.9312, 337.6444)
  line L690 (640.9312, 337.6444) -> (641.074, 337.467)
  line L691 (641.074, 337.467) -> (641.2513, 337.3173)
  line L692 (641.2513, 337.3173) -> (641.4497, 337.221)
  line L693 (641.4497, 337.221) -> (641.6459, 337.2855)
  line L694 (641.6459, 337.2855) -> (641.7783, 337.4818)
  line L695 (641.7783, 337.4818) -> (641.7901, 337.7652)
  line L696 (641.7901, 337.7652) -> (641.6541, 338.0807)
  line L697 (641.6541, 338.0807) -> (641.4196, 338.3328)
  line L698 (641.4196, 338.3328) -> (641.359, 338.4957)
  line L699 (641.359, 338.4957) -> (641.5219, 338.6755)
  line L700 (641.5219, 338.6755) -> (641.6875, 338.8527)
  line L701 (641.6875, 338.8527) -> (641.8397, 339.012)
  line L702 (641.8397, 339.012) -> (641.9195, 339.164)
  line L703 (641.9195, 339.164) -> (641.91, 339.3267)
  line L704 (641.91, 339.3267) -> (641.8249, 339.4845)
  line L705 (641.8249, 339.4845) -> (641.8179, 339.6062)
  line L706 (641.8179, 339.6062) -> (641.8756, 339.7158)
  line L707 (641.8756, 339.7158) -> (641.9948, 339.8783)
  line L708 (641.9948, 339.8783) -> (642.1243, 340.1092)
  line L709 (642.1243, 340.1092) -> (642.1842, 340.3675)
  line L710 (642.1842, 340.3675) -> (642.1632, 340.876)
  line L711 (642.1632, 340.876) -> (642.4317, 341.3803)
  line L712 (642.4317, 341.3803) -> (643.0116, 341.5945)
  line L713 (643.0116, 341.5945) -> (643.662, 341.6192)
  line L714 (643.662, 341.6192) -> (644.1803, 341.6752)
  line L715 (644.1803, 341.6752) -> (644.6825, 341.7873)
  line L716 (644.6825, 341.7873) -> (645.1009, 341.94)
  line L717 (645.1009, 341.94) -> (645.2923, 342.2013)
  line L718 (645.2923, 342.2013) -> (645.2999, 342.5311)
  line L719 (645.2999, 342.5311) -> (645.1703, 342.8111)
  line L720 (645.1703, 342.8111) -> (645.0727, 343.0529)
  line L721 (645.0727, 343.0529) -> (645.0009, 343.307)
  line L722 (645.0009, 343.307) -> (644.9495, 343.5589)
  line L723 (644.9495, 343.5589) -> (644.9292, 343.8126)
  line L724 (644.9292, 343.8126) -> (644.9075, 344.0655)
  line L725 (644.9075, 344.0655) -> (644.8528, 344.2885)
  line L726 (644.8528, 344.2885) -> (644.7662, 344.4784)
  line L727 (644.7662, 344.4784) -> (644.6518, 344.6546)
  line L728 (644.6518, 344.6546) -> (644.5158, 344.8274)
  line L729 (644.5158, 344.8274) -> (644.4573, 345.0121)
  line L730 (644.4573, 345.0121) -> (644.4937, 345.193)
  line L731 (644.4937, 345.193) -> (644.681, 345.4942)
  line L732 (644.681, 345.4942) -> (645.0696, 345.8439)
  line L733 (645.0696, 345.8439) -> (645.5473, 346.0497)
  line L734 (645.5473, 346.0497) -> (646.292, 346.1333)
  line L735 (646.292, 346.1333) -> (647.2654, 345.9804)
  line L736 (647.2654, 345.9804) -> (648.181, 345.6131)
  line L737 (648.181, 345.6131) -> (649.162, 345.0699)
  line L738 (649.162, 345.0699) -> (650.2162, 344.352)
  line L739 (650.2162, 344.352) -> (651.156, 343.4951)
  line L740 (651.156, 343.4951) -> (651.8587, 342.5889)
  line L741 (651.8587, 342.5889) -> (652.3075, 341.7803)
  line L742 (652.3075, 341.7803) -> (652.6357, 340.9186)
  line L743 (652.6357, 340.9186) -> (652.8597, 339.9664)
  line L744 (652.8597, 339.9664) -> (653.0795, 338.9452)
  line L745 (653.0795, 338.9452) -> (653.2815, 337.921)
  line L746 (653.2815, 337.921) -> (653.4749, 336.6266)
  line L747 (653.4749, 336.6266) -> (653.6329, 334.9303)
  line L748 (653.6329, 334.9303) -> (653.64, 333.2269)
  line L749 (653.64, 333.2269) -> (653.5125, 331.9053)
  line L750 (653.5125, 331.9053) -> (653.4527, 331.1762)
  line L751 (653.4527, 331.1762) -> (653.4097, 330.445)
  line L752 (653.4097, 330.445) -> (653.3768, 329.9973)
  line L753 (653.3768, 329.9973) -> (653.341, 329.9847)
  line L754 (653.341, 329.9847) -> (653.3006, 329.9705)
  line L755 (653.3006, 329.9705) -> (653.2343, 330.0785)
  line L756 (653.2343, 330.0785) -> (653.0864, 330.3682)
  line L757 (653.0864, 330.3682) -> (652.9397, 330.6585)
  line L758 (652.9397, 330.6585) -> (652.5578, 331.4365)
  line L759 (652.5578, 331.4365) -> (651.7302, 332.977)
  line L760 (651.7302, 332.977) -> (650.7272, 334.4004)
  line L761 (650.7272, 334.4004) -> (649.6787, 335.4361)
  line L762 (649.6787, 335.4361) -> (648.9013, 336.0163)
  line L763 (648.9013, 336.0163) -> (648.0503, 336.4816)
  line L764 (648.0503, 336.4816) -> (647.2286, 336.7737)
  line L765 (647.2286, 336.7737) -> (646.5919, 336.9521)
  line L766 (646.5919, 336.9521) -> (645.9486, 337.0788)
  line L767 (645.9486, 337.0788) -> (645.3737, 337.118)
  line L768 (645.3737, 337.118) -> (644.935, 337.0846)
  line L769 (644.935, 337.0846) -> (644.4965, 337.0158)
  line L770 (644.4965, 337.0158) -> (644.0896, 336.9396)
  line L771 (644.0896, 336.9396) -> (643.7371, 336.8506)
  line L772 (643.7371, 336.8506) -> (643.3867, 336.7494)
  line L773 (643.3867, 336.7494) -> (642.9684, 336.6283)
  line L774 (642.9684, 336.6283) -> (642.4606, 336.4025)
  line L775 (642.4606, 336.4025) -> (641.9974, 336.1008)
  line L776 (641.9974, 336.1008) -> (641.4154, 335.5958)
  line L777 (641.4154, 335.5958) -> (640.6559, 334.7195)
  line L778 (640.6559, 334.7195) -> (640.0496, 333.7342)
  line L779 (640.0496, 333.7342) -> (639.598, 332.6628)
  line L780 (639.598, 332.6628) -> (639.4033, 331.5928)
  line L781 (639.4033, 331.5928) -> (639.5285, 330.5297)
  line L782 (639.5285, 330.5297) -> (639.9163, 329.6261)
  line L783 (639.9163, 329.6261) -> (640.2591, 329.0578)
  line L784 (640.2591, 329.0578) -> (640.7016, 328.5777)
  line L785 (640.7016, 328.5777) -> (641.3259, 328.2297)
  line L786 (641.3259, 328.2297) -> (642.0543, 327.9898)
  line L787 (642.0543, 327.9898) -> (642.8045, 327.9153)
  line L788 (642.8045, 327.9153) -> (643.4239, 328.0198)
  line L789 (643.4239, 328.0198) -> (643.7234, 328.164)
  line L790 (643.7234, 328.164) -> (644.0036, 328.3597)
  line L791 (644.0036, 328.3597) -> (644.2303, 328.545)
  line L792 (644.2303, 328.545) -> (644.3579, 328.5949)
  line L793 (644.3579, 328.5949) -> (644.4647, 328.5515)
  line L794 (644.4647, 328.5515) -> (644.6078, 328.5483)
  line L795 (644.6078, 328.5483) -> (644.8137, 328.7622)
  line L796 (644.8137, 328.7622) -> (645.0075, 328.9633)
  line L797 (645.0075, 328.9633) -> (645.2007, 329.0779)
  line L798 (645.2007, 329.0779) -> (645.4102, 329.0354)
  line L799 (645.4102, 329.0354) -> (645.6024, 328.9962)
  line L800 (645.6024, 328.9962) -> (645.775, 329.1124)
  line L801 (645.775, 329.1124) -> (645.9143, 329.5669)
  line L802 (645.9143, 329.5669) -> (646.0494, 330.0046)
  line L803 (646.0494, 330.0046) -> (646.1598, 330.3696)
  line L804 (646.1598, 330.3696) -> (646.1419, 330.5458)
  line L805 (646.1419, 330.5458) -> (646.04, 330.6792)
  line L806 (646.04, 330.6792) -> (645.7833, 330.864)
  line L807 (645.7833, 330.864) -> (645.4962, 331.381)
  line L808 (645.4962, 331.381) -> (645.5693, 331.9567)
  line L809 (645.5693, 331.9567) -> (645.9469, 332.3437)
  line L810 (645.9469, 332.3437) -> (646.3957, 332.4185)
  line L811 (646.3957, 332.4185) -> (646.8578, 332.3259)
  line L812 (646.8578, 332.3259) -> (647.1637, 332.0494)
  line L813 (647.1637, 332.0494) -> (647.2902, 331.5479)
  line L814 (647.2902, 331.5479) -> (647.1838, 331.048)
  line L815 (647.1838, 331.048) -> (646.9158, 330.7499)
  line L816 (646.9158, 330.7499) -> (646.8237, 330.6249)
  line L817 (646.8237, 330.6249) -> (646.8245, 330.496)
  line L818 (646.8245, 330.496) -> (646.909, 330.2956)
  line L819 (646.909, 330.2956) -> (647.078, 329.9354)
  line L820 (647.078, 329.9354) -> (647.2514, 329.5773)
  line L821 (647.2514, 329.5773) -> (647.4089, 329.2696)
  line L822 (647.4089, 329.2696) -> (647.5223, 329.1487)
  line L823 (647.5223, 329.1487) -> (647.6603, 329.1508)
  line L824 (647.6603, 329.1508) -> (647.8084, 329.2959)
  line L825 (647.8084, 329.2959) -> (647.9268, 329.3852)
  line L826 (647.9268, 329.3852) -> (648.0544, 329.3725)
  line L827 (648.0544, 329.3725) -> (648.1713, 329.2651)
  line L828 (648.1713, 329.2651) -> (648.2406, 329.2248)
  line L829 (648.2406, 329.2248) -> (648.3206, 329.1923)
  line L830 (648.3206, 329.1923) -> (648.4374, 329.1145)
  line L831 (648.4374, 329.1145) -> (648.6695, 329.026)
  line L832 (648.6695, 329.026) -> (648.8857, 329.0926)
  line L833 (648.8857, 329.0926) -> (649.1375, 329.3402)
  line L834 (649.1375, 329.3402) -> (649.338, 329.6124)
  line L835 (649.338, 329.6124) -> (649.2845, 329.8203)
  line L836 (649.2845, 329.8203) -> (648.9894, 330.1015)
  line L837 (648.9894, 330.1015) -> (648.8461, 330.3743)
  line L838 (648.8461, 330.3743) -> (648.8467, 330.6597)
  line L839 (648.8467, 330.6597) -> (648.9019, 330.9534)
  line L840 (648.9019, 330.9534) -> (649.0437, 331.1526)
  line L841 (649.0437, 331.1526) -> (649.2599, 331.256)
  line L842 (649.2599, 331.256) -> (649.5081, 331.3325)
  line L843 (649.5081, 331.3325) -> (649.7429, 331.4624)
  line L844 (649.7429, 331.4624) -> (649.8689, 331.644)
  line L845 (649.8689, 331.644) -> (649.8709, 331.9244)
  line L846 (649.8709, 331.9244) -> (649.7689, 332.2531)
  line L847 (649.7689, 332.2531) -> (649.5634, 332.4074)
  line L848 (649.5634, 332.4074) -> (649.1862, 332.4392)
  line L849 (649.1862, 332.4392) -> (648.8348, 332.4703)
  line L850 (648.8348, 332.4703) -> (648.6591, 332.6342)
  line L851 (648.6591, 332.6342) -> (648.5396, 332.9759)
  line L852 (648.5396, 332.9759) -> (648.5396, 333.1972)
  line L853 (648.5396, 333.1972) -> (648.5993, 333.4307)
  line L854 (648.5993, 333.4307) -> (648.6908, 333.6545)
  line L855 (648.6908, 333.6545) -> (648.7603, 333.8764)
  line L856 (648.7603, 333.8764) -> (648.7114, 334.0594)
  line L857 (648.7114, 334.0594) -> (648.5368, 334.1793)
  line L858 (648.5368, 334.1793) -> (648.5255, 334.1971)
  line L859 (648.5255, 334.1971) -> (648.4352, 334.2619)
  line L860 (648.4352, 334.2619) -> (648.1296, 334.43)
  line L861 (648.1296, 334.43) -> (647.8956, 334.3619)
  line L862 (647.8956, 334.3619) -> (647.5624, 334.0726)
  line L863 (647.5624, 334.0726) -> (647.1848, 333.9698)
  line L864 (647.1848, 333.9698) -> (646.8096, 334.0976)
  line L865 (646.8096, 334.0976) -> (646.6055, 334.3548)
  line L866 (646.6055, 334.3548) -> (646.5912, 334.3837)
  line L867 (646.5912, 334.3837) -> (646.5764, 334.4123)
  line L868 (646.5764, 334.4123) -> (646.5328, 334.5402)
  line L869 (646.5328, 334.5402) -> (646.36, 334.9153)
  line L870 (646.36, 334.9153) -> (646.1032, 335.0114)
  line L871 (646.1032, 335.0114) -> (645.6643, 334.9395)